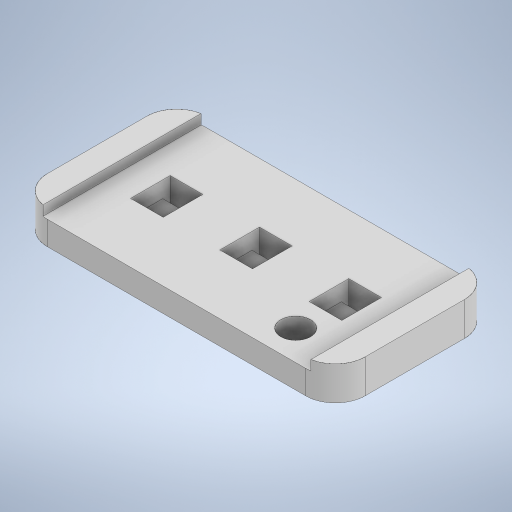
# Autodesk Inventor part: button_bottom
Saved by Autodesk Inventor 2024.3 (Build 283343000, 343)
## iProperties
Created: 2025-07-27
Part Number: button_bottom
Material: Ogólny
Document SubType Name: Modeling
Designer: User
Density: 1 g/cm^3
Appearance: Domyślna
Author: User
Autodesk Inventor part; units mm, degrees
ref_plane "YZ Plane" through (0, 0, 0) normal (1, 0, 0) x (0, 1, 0)
ref_plane "XZ Plane" through (0, 0, 0) normal (0, 1, 0) x (-1, 0, 0)
ref_plane "XY Plane" through (0, 0, 0) normal (0, 0, 1) x (1, 0, 0)
sketch "Szkic1" plane through (0, 0, 0) normal (0, 1, 0) x (-1, 0, 0)
  line L0 (0, 0) -> (54, 0)
  line L1 (54, 0) -> (54, -32)
  line L2 (54, -32) -> (0, -32)
  line L3 (0, -32) -> (0, 0)
  line L4 (54, 0) -> (0, 0)
  line L5 (54, 0) -> (36, 0)
  line L6 (36, 0) -> (18, 0)
  line L7 (18, 0) -> (0, 0)
  line L8 (54, -16) -> (0, -16)
  line L9 (41.7, -12) -> (48.3, -12)
  line L10 (48.3, -12) -> (48.3, -20)
  line L11 (48.3, -20) -> (41.7, -20)
  line L12 (41.7, -20) -> (41.7, -12)
  line L13 (41.7, -12) -> (48.3, -20) construction
  line L14 (48.3, -12) -> (41.7, -20) construction
  line L15 (23.7, -12) -> (30.3, -12)
  line L16 (30.3, -12) -> (30.3, -20)
  line L17 (30.3, -20) -> (23.7, -20)
  line L18 (23.7, -20) -> (23.7, -12)
  line L19 (5.7, -12) -> (12.3, -12)
  line L20 (12.3, -12) -> (12.3, -20)
  line L21 (12.3, -20) -> (5.7, -20)
  line L22 (5.7, -20) -> (5.7, -12)
  line L23 (48.3, -12) -> (41.7, -12)
  line L24 (41.7, -12) -> (41.7, -13.5)
  line L25 (41.7, -13.5) -> (48.3, -13.5)
  line L26 (48.3, -13.5) -> (48.3, -12)
  line L27 (48.3, -20) -> (41.7, -20)
  line L28 (41.7, -20) -> (41.7, -18.5)
  line L29 (41.7, -18.5) -> (48.3, -18.5)
  line L30 (48.3, -18.5) -> (48.3, -20)
  line L31 (12.3, -12) -> (12.3, -20)
  line L32 (23.7, -18.5) -> (30.3, -18.5)
  line L33 (23.7, -13.5) -> (30.3, -13.5)
  line L34 (-5.7, -12) -> (-5.7, -20)
  line L35 (5.7, -18.5) -> (12.3, -18.5)
  line L36 (5.7, -13.5) -> (12.3, -13.5)
  point P0 (45, -16)
  point P1 (12.3, -18.5)
  dimension "d0" = 54
  dimension "d1" = 32
  dimension "d2" = 18
  dimension "d3" = 18
  dimension "d4" = 6.6
  dimension "d5" = 8
  dimension "d6" = 9
  dimension "d9" = 18
  dimension "d18" = 1.5
  dimension "d19" = 1.5
  dimension "d22" = 18
  constraints: 74 end point, 9 equal length, 6 horizontal, 5 perpendicular, 5 point on line, 4 midpoint, 34 other
  measures "d0" distance of L1.end L2.end
  measures "d1" distance of L0.end L1.end
  measures "d2" distance of L0.end L5.end
  measures "d3" distance of L5.end L6.end
  measures "d4" distance of L10.end L11.end
  measures "d5" distance of L9.end L10.end
  measures "d6" distance of L8.start point (45, -16)
  measures "d9" distance of L9.start L15.start
  measures "d18" distance of L24.end L23.end
  measures "d19" distance of L27.end L28.end
  measures "d22" distance of L15.end L31.start
extrude "Wyciągnięcie proste1" add sketch "Szkic1" along normal blind 1 and the other way blind 2
extrude "Wyciągnięcie proste2" cut sketch "Szkic1" along normal blind 4.75 and the other way blind 5 contours L35 L20 L21 L22 | L22 L19 L20 L36 | L32 L16 L17 L18 | L18 L15 L16 L33 | L25 L12 L9 L10 | L10 L11 L12 L29
extrude "Wyciągnięcie proste3" cut sketch "Szkic1" along normal blind 1 and the other way blind 0.5 contours L22 L36 L20 L8 | L8 L20 L35 L22 | L18 L33 L16 L8 | L8 L16 L32 L18 | L10 L29 L12 L8 | L8 L12 L25 L10
move faces "Przesuń1" translate (0, 1.5, 0) faces at (-25.9, 1, -28)
sketch "Szkic2" plane through (0, -2, 0) normal (0, -1, 0) x (1, 0, 0)
  line L0 (0, -32) -> (0, 0) projected
  circle A0 centre (2.1999, -26.0004) radius 1.7
  line L1 (0, 0) -> (5, 0)
  line L2 (5, 0) -> (5, -32)
  line L3 (5, -32) -> (0, -32)
  line L4 (0, -32) -> (0, 0)
  line L5 (0, 0) -> (-54, 0) projected
  line L6 (-27, 0) -> (-27, -32)
  line L7 (-54, -32) -> (0, -32) projected
  line L8 (-54, -32) -> (-54, 0)
  line L9 (-54, 0) -> (-59, 0)
  line L10 (-59, 0) -> (-59, -32)
  line L11 (-59, -32) -> (-54, -32)
  line L12 (-54, -32) -> (-54, 0)
  line L13 (0, -16) -> (5, -16)
  line L14 (2.2, -16) -> (2.2, -26)
  line L15 (2.2, -16) -> (12.2, -16) construction
  circle A1 centre (2.1999, -5.9996) radius 1.7
  circle A2 centre (-56.1999, -26.0004) radius 1.7
  circle A3 centre (-56.1999, -5.9996) radius 1.7
  dimension "d39" = 3.4
  dimension "d40" = 5
  dimension "d59" = 10
  dimension "d60" = 90
  dimension "d61" = 2.8001
  constraints: 26 end point, 7 symmetric about line, 4 centre point, 4 midpoint, 3 perpendicular, 2 horizontal, 2 parallel, 1 vertical, 3 other
  measures "d39" diameter of A0
  measures "d40" distance of L2.end L3.end
  measures "d59" distance of L14.start L14.end
  measures "d60" angle of L14 L15
  measures "d61" distance from line of A0.centre L2
extrude "Wyciągnięcie proste4" add sketch "Szkic2" against normal blind 3 contours L0 L13 L2 L3 | L0 L1 L2 L13 | L11 L10 L9 L8
fillet "Zaokrąglenie1" radius 6 4 edges at (-59, -0.5, 0) (5, -0.5, 0) (5, -0.5, -32) (-59, -0.5, -32)
sketch "Szkic3" plane through (-53, 2.5, 0) normal (0, 1, 0) x (1, 0, 0)
  line L0 (47.3, 12) -> (40.7, 12) projected
  line L1 (44, 12) -> (44, 6)
  circle A0 centre (44, 6) radius 3
  point P0 (53, 0)
  dimension "d44" = 6
  dimension "d45" = 6
  constraints: 2 end point, 1 centre point, 1 coincident, 1 midpoint, 1 vertical
  measures "d44" distance of L1.start L1.end
  measures "d45" diameter of A0
extrude "Wyciągnięcie proste5" cut sketch "Szkic3" against normal blind 11.5
move faces "Przesuń2" translate (0, 0.3, 0) faces at (-28.1, 2.5, -28)
sketch "Szkic4" plane through (0, 1, 0) normal (0, 1, 0) x (1, 0, 0)
  line L0 (5, 26) -> (5, 6) projected
  line L1 (-53, 32) -> (-1, 32) projected
  arc A0 (5, 26) -> (-1, 32) centre (-1, 26) ccw
  arc A1 (-1, 0) -> (0, 0.0839) centre (-1, 6) ccw projected
  arc A2 (0, 0.0839) -> (5, 6) centre (-1, 6) ccw projected
  arc A3 (0, 0.0839) -> (5, 6) centre (-1, 6) ccw
  line L2 (5, 26) -> (5, 6)
  line L3 (0, 0.0839) -> (0, 31.9161) projected
  line L4 (0, 0.0839) -> (0, 31.9161)
  line L5 (-27, 32) -> (-27, 0.0839)
  line L6 (-59, 26) -> (-59, 6)
  line L7 (-1, 32) -> (-53, 32)
  arc A4 (-53, 32) -> (-59, 26) centre (-53, 26) ccw
  arc A5 (-54, 0.0839) -> (-53, 0) centre (-53, 6) ccw
  arc A6 (-59, 6) -> (-54, 0.0839) centre (-53, 6) ccw
  arc A7 (-59, 6) -> (-54, 0.0839) centre (-53, 6) ccw
  line L8 (-59, 26) -> (-59, 6)
  line L9 (-54, 0.0839) -> (-54, 31.9161)
  line L10 (-54, 0.0839) -> (-54, 31.9161)
  point P0 (0, 0)
  point P1 (-54, 0)
  constraints: 16 end point, 12 point on circle, 12 symmetric about line, 6 centre point, 2 collinear, 1 midpoint, 1 vertical, 4 other
extrude "Wyciągnięcie proste6" add sketch "Szkic4" along normal up to surface (1.8 mm away)
sketch "Szkic5" plane through (0, -2, 0) normal (0, -1, 0) x (1, 0, 0)
  circle A0 centre (2.1999, -26.0004) radius 1.7 projected
  circle A1 centre (2.1999, -26.0004) radius 2.1
  circle A2 centre (-56.1999, -5.9996) radius 1.7 projected
  circle A3 centre (-56.1999, -5.9996) radius 2.1
  circle A4 centre (-56.1999, -26.0004) radius 1.7 projected
  circle A5 centre (-56.1999, -26.0004) radius 2.1
  circle A6 centre (2.1999, -5.9996) radius 1.7 projected
  circle A7 centre (2.1999, -5.9996) radius 2.1
  point P0 (0, 0)
  point P1 (-56, -16)
  dimension "d55" = 4.2
  dimension "d62" = 4.2
  dimension "d63" = 4.2
  dimension "d64" = 4.2
  constraints: 4 centre point, 4 coincident
  measures "d55" diameter of A1
  measures "d62" diameter of A3
  measures "d63" diameter of A5
  measures "d64" diameter of A7
extrude "Wyciągnięcie proste7" cut sketch "Szkic5" against normal blind 1
sketch "Szkic6" plane through (-53, 2.8, 0) normal (0, 1, 0) x (1, 0, 0)
  line L0 (26, 32) -> (26, 0)
  line L1 (53, 0) -> (-1, 0)
  line L2 (-1, 0) -> (-1, 32)
  line L3 (-1, 32) -> (53, 32)
  line L4 (53, 32) -> (53, 0)
  line L5 (53, 0) -> (-1, 32) construction
  line L6 (-1, 0) -> (53, 32) construction
  arc A0 (0, 32) -> (-6, 26) centre (0, 26) ccw projected
  arc A1 (0, 32) -> (-6, 26) centre (0, 26) ccw
  arc A2 (-6, 6) -> (0, 0) centre (0, 6) ccw projected
  arc A3 (-6, 6) -> (0, 0) centre (0, 6) ccw
  line L7 (-1, 0) -> (-1, 32)
  line L8 (-6, 6) -> (-6, 26) projected
  line L9 (-6, 6) -> (-6, 26)
  line L10 (53, 0) -> (53, 32)
  arc A4 (58, 26) -> (52, 32) centre (52, 26) ccw
  arc A5 (52, 0) -> (58, 6) centre (52, 6) ccw
  line L11 (53, 0) -> (53, 32)
  line L12 (58, 6) -> (58, 26)
  line L13 (58, 6) -> (58, 26)
  point P0 (52, 32)
  point P1 (26, 16)
  point P2 (53, 31.9161)
  point P3 (53, 0.0839)
  point P4 (-1, 0.0839)
  point P5 (-1, 31.9161)
  dimension "d69" = 54
  dimension "d70" = 32
  constraints: 26 end point, 10 point on circle, 7 symmetric about line, 4 centre point, 3 midpoint, 3 parallel, 1 collinear, 1 horizontal, 1 perpendicular, 2 other
  measures "d69" distance of L2.end L3.end
  measures "d70" distance of L1.end L2.end
extrude "Wyciągnięcie proste8" add sketch "Szkic6" along normal blind 2 contours L2 A2 L8 A0 | A4 L12 A5 L4
move faces "Przesuń3" translate (0, 2, 0) faces at (-56.1316, 1, -25.5032) (-55.2529, 1, -5.5604) (1.8945, 1, -25.3984) (2.7017, 1, -5.7363)
